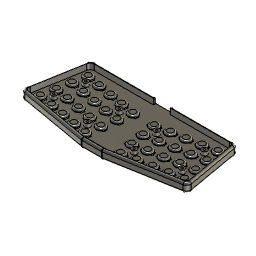
pusheenz40 low tolerance v2 v8 (Autodesk Fusion 360 design; units mm, degrees)
Autodesk Fusion 360 part; units mm, degrees
note: some values were not read from the file. Chosen so that the rebuilt part matches the saved one: which bodies a step acts on. Set by a fixed rule: which sketch regions a step uses.
(part 1 of 2)
sketch "Sketch1" plane through (0, 0, 0) normal (0, 0, 1) x (1, 0, 0)
  line L0 (-7.5882, -2.7237) -> (-0.9058, 35.1744)
  line L1 (2.0486, 37.6534) -> (102.6819, 37.6534)
  line L2 (105.6363, 35.1744) -> (112.3188, -2.7237)
  line L3 (109.8853, -6.1991) -> (59.9186, -15.0095)
  line L4 (59.3977, -15.0551) -> (45.3329, -15.0551)
  line L5 (44.8119, -15.0095) -> (-5.1548, -6.1991)
  arc A0 (2.0486, 37.6534) -> (-0.9058, 35.1744) centre (2.0486, 34.6534) ccw
  arc A1 (105.6363, 35.1744) -> (102.6819, 37.6534) centre (102.6819, 34.6534) ccw
  arc A2 (109.8853, -6.1991) -> (112.3188, -2.7237) centre (109.3644, -3.2446) ccw
  arc A3 (59.3977, -15.0551) -> (59.9186, -15.0095) centre (59.3977, -12.0551) ccw
  arc A4 (44.8119, -15.0095) -> (45.3329, -15.0551) centre (45.3329, -12.0551) ccw
  arc A5 (-7.5882, -2.7237) -> (-5.1548, -6.1991) centre (-4.6338, -3.2446) ccw
  line L6 (-5.8506, -1.507) -> (0.3109, 33.4367)
  line L7 (3.2654, 35.9157) -> (101.4652, 35.9157)
  line L8 (104.4196, 33.4367) -> (110.5811, -1.507)
  line L9 (108.1476, -4.9823) -> (61.1353, -13.2719)
  line L10 (60.6144, -13.3174) -> (44.1162, -13.3174)
  line L11 (43.5952, -13.2719) -> (-3.4171, -4.9823)
  arc A6 (3.2654, 35.9157) -> (0.3109, 33.4367) centre (3.2654, 32.9157) ccw
  arc A7 (104.4196, 33.4367) -> (101.4652, 35.9157) centre (101.4652, 32.9157) ccw
  arc A8 (108.1476, -4.9823) -> (110.5811, -1.507) centre (107.6267, -2.0279) ccw
  arc A9 (60.6144, -13.3174) -> (61.1353, -13.2719) centre (60.6144, -10.3174) ccw
  arc A10 (43.5952, -13.2719) -> (44.1162, -13.3174) centre (44.1162, -10.3174) ccw
  arc A11 (-5.8506, -1.507) -> (-3.4171, -4.9823) centre (-2.8961, -2.0279) ccw
  line L12 (-5.2713, -1.1014) -> (0.7165, 32.8575)
  line L13 (3.6709, 35.3365) -> (101.0596, 35.3365)
  line L14 (104.014, 32.8575) -> (110.0019, -1.1014)
  line L15 (107.5684, -4.5767) -> (61.5409, -12.6926)
  line L16 (61.02, -12.7382) -> (43.7106, -12.7382)
  line L17 (43.1896, -12.6926) -> (-2.8379, -4.5767)
  arc A12 (3.6709, 35.3365) -> (0.7165, 32.8575) centre (3.6709, 32.3365) ccw
  arc A13 (104.014, 32.8575) -> (101.0596, 35.3365) centre (101.0596, 32.3365) ccw
  arc A14 (107.5684, -4.5767) -> (110.0019, -1.1014) centre (107.0475, -1.6223) ccw
  arc A15 (61.02, -12.7382) -> (61.5409, -12.6926) centre (61.02, -9.7382) ccw
  arc A16 (43.1896, -12.6926) -> (43.7106, -12.7382) centre (43.7106, -9.7382) ccw
  arc A17 (-5.2713, -1.1014) -> (-2.8379, -4.5767) centre (-2.3169, -1.6223) ccw
  line L18 (-3.6888, -0.8219) -> (-3.3564, -0.8805)
  line L19 (2.8528, -1.9754) -> (3.1852, -2.034)
  arc A18 (3.1852, -2.034) -> (3.7644, -1.6284) centre (3.272, -1.5416) ccw
  line L20 (3.7644, -1.6284) -> (4.0943, 0.2427)
  arc A19 (4.0943, 0.2427) -> (3.6888, 0.8219) centre (3.6019, 0.3295) ccw
  line L21 (3.6888, 0.8219) -> (3.3564, 0.8805)
  line L22 (-2.8528, 1.9754) -> (-3.1852, 2.034)
  arc A20 (-3.1852, 2.034) -> (-3.7644, 1.6284) centre (-3.272, 1.5416) ccw
  line L23 (-3.7644, 1.6284) -> (-4.0943, -0.2427)
  arc A21 (-4.0943, -0.2427) -> (-3.6888, -0.8219) centre (-3.6019, -0.3295) ccw
  line L24 (-1.9523, 9.0261) -> (-1.6199, 8.9675)
  line L25 (4.5893, 7.8727) -> (4.9217, 7.8141)
  arc A22 (4.9217, 7.8141) -> (5.5009, 8.2197) centre (5.0085, 8.3065) ccw
  line L26 (5.5009, 8.2197) -> (5.8308, 10.0908)
  arc A23 (5.8308, 10.0908) -> (5.4253, 10.67) centre (5.3384, 10.1776) ccw
  line L27 (5.4253, 10.67) -> (5.0929, 10.7286)
  line L28 (-1.1164, 11.8235) -> (-1.4487, 11.8821)
  arc A24 (-1.4487, 11.8821) -> (-2.0279, 11.4765) centre (-1.5355, 11.3897) ccw
  line L29 (-2.0279, 11.4765) -> (-2.3579, 9.6054)
  arc A25 (-2.3579, 9.6054) -> (-1.9523, 9.0261) centre (-1.8655, 9.5185) ccw
  line L30 (-0.2158, 18.8742) -> (0.1165, 18.8156)
  line L31 (6.3258, 17.7208) -> (6.6582, 17.6622)
  arc A26 (6.6582, 17.6622) -> (7.2374, 18.0677) centre (6.745, 18.1546) ccw
  line L32 (7.2374, 18.0677) -> (7.5673, 19.9389)
  arc A27 (7.5673, 19.9389) -> (7.1617, 20.5181) centre (7.0749, 20.0257) ccw
  line L33 (7.1617, 20.5181) -> (6.8294, 20.5767)
  line L34 (0.6201, 21.6716) -> (0.2878, 21.7302)
  arc A28 (0.2878, 21.7302) -> (-0.2915, 21.3246) centre (0.201, 21.2378) ccw
  line L35 (-0.2915, 21.3246) -> (-0.6214, 19.4534)
  arc A29 (-0.6214, 19.4534) -> (-0.2158, 18.8742) centre (-0.129, 19.3666) ccw
  line L36 (1.5207, 28.7223) -> (1.853, 28.6637)
  line L37 (8.0623, 27.5688) -> (8.3946, 27.5102)
  arc A30 (8.3946, 27.5102) -> (8.9739, 27.9158) centre (8.4815, 28.0026) ccw
  line L38 (8.9739, 27.9158) -> (9.3038, 29.7869)
  arc A31 (9.3038, 29.7869) -> (8.8982, 30.3662) centre (8.8114, 29.8738) ccw
  line L39 (8.8982, 30.3662) -> (8.5659, 30.4248)
  line L40 (2.3566, 31.5196) -> (2.0243, 31.5782)
  arc A32 (2.0243, 31.5782) -> (1.445, 31.1727) centre (1.9374, 31.0858) ccw
  line L41 (1.445, 31.1727) -> (1.1151, 29.3015)
  arc A33 (1.1151, 29.3015) -> (1.5207, 28.7223) centre (1.6075, 29.2147) ccw
  line L42 (6.1593, -2.5584) -> (6.4917, -2.617)
  line L43 (12.7009, -3.7119) -> (13.0333, -3.7705)
  arc A34 (13.0333, -3.7705) -> (13.6125, -3.3649) centre (13.1201, -3.2781) ccw
  line L44 (13.6125, -3.3649) -> (13.9424, -1.4938)
  arc A35 (13.9424, -1.4938) -> (13.5368, -0.9145) centre (13.45, -1.4069) ccw
  line L45 (13.5368, -0.9145) -> (13.2045, -0.8559)
  line L46 (6.9952, 0.2389) -> (6.6629, 0.2975)
  arc A36 (6.6629, 0.2975) -> (6.0837, -0.1081) centre (6.5761, -0.1949) ccw
  line L47 (6.0837, -0.1081) -> (5.7537, -1.9792)
  arc A37 (5.7537, -1.9792) -> (6.1593, -2.5584) centre (6.2461, -2.066) ccw
  line L48 (7.8958, 7.2897) -> (8.2281, 7.2311)
  line L49 (14.4374, 6.1362) -> (14.7697, 6.0776)
  arc A38 (14.7697, 6.0776) -> (15.349, 6.4832) centre (14.8566, 6.57) ccw
  line L50 (15.349, 6.4832) -> (15.6789, 8.3543)
  arc A39 (15.6789, 8.3543) -> (15.2733, 8.9335) centre (15.1865, 8.4411) ccw
  line L51 (15.2733, 8.9335) -> (14.941, 8.9921)
  line L52 (8.7317, 10.087) -> (8.3994, 10.1456)
  arc A40 (8.3994, 10.1456) -> (7.8201, 9.74) centre (8.3125, 9.6532) ccw
  line L53 (7.8201, 9.74) -> (7.4902, 7.8689)
  arc A41 (7.4902, 7.8689) -> (7.8958, 7.2897) centre (7.9826, 7.7821) ccw
  line L54 (9.6323, 17.1377) -> (9.9646, 17.0791)
  line L55 (16.1739, 15.9843) -> (16.5062, 15.9257)
  arc A42 (16.5062, 15.9257) -> (17.0855, 16.3312) centre (16.5931, 16.4181) ccw
  line L56 (17.0855, 16.3312) -> (17.4154, 18.2024)
  arc A43 (17.4154, 18.2024) -> (17.0098, 18.7816) centre (16.923, 18.2892) ccw
  line L57 (17.0098, 18.7816) -> (16.6775, 18.8402)
  line L58 (10.4682, 19.9351) -> (10.1359, 19.9937)
  arc A44 (10.1359, 19.9937) -> (9.5566, 19.5881) centre (10.049, 19.5013) ccw
  line L59 (9.5566, 19.5881) -> (9.2267, 17.717)
  arc A45 (9.2267, 17.717) -> (9.6323, 17.1377) centre (9.7191, 17.6301) ccw
  line L60 (11.3688, 26.9858) -> (11.7011, 26.9272)
  line L61 (17.9104, 25.8323) -> (18.2427, 25.7737)
  arc A46 (18.2427, 25.7737) -> (18.8219, 26.1793) centre (18.3295, 26.2662) ccw
  line L62 (18.8219, 26.1793) -> (19.1519, 28.0505)
  arc A47 (19.1519, 28.0505) -> (18.7463, 28.6297) centre (18.6595, 28.1373) ccw
  line L63 (18.7463, 28.6297) -> (18.4139, 28.6883)
  line L64 (12.2047, 29.7832) -> (11.8723, 29.8418)
  arc A48 (11.8723, 29.8418) -> (11.2931, 29.4362) centre (11.7855, 29.3494) ccw
  line L65 (11.2931, 29.4362) -> (10.9632, 27.565)
  arc A49 (10.9632, 27.565) -> (11.3688, 26.9858) centre (11.4556, 27.4782) ccw
  line L66 (16.0074, -4.2949) -> (16.3397, -4.3535)
  line L67 (22.549, -5.4484) -> (22.8813, -5.507)
  arc A50 (22.8813, -5.507) -> (23.4606, -5.1014) centre (22.9682, -5.0146) ccw
  line L68 (23.4606, -5.1014) -> (23.7905, -3.2303)
  arc A51 (23.7905, -3.2303) -> (23.3849, -2.651) centre (23.2981, -3.1434) ccw
  line L69 (23.3849, -2.651) -> (23.0526, -2.5924)
  line L70 (16.8433, -1.4976) -> (16.511, -1.439)
  arc A52 (16.511, -1.439) -> (15.9317, -1.8445) centre (16.4241, -1.9314) ccw
  line L71 (15.9317, -1.8445) -> (15.6018, -3.7157)
  arc A53 (15.6018, -3.7157) -> (16.0074, -4.2949) centre (16.0942, -3.8025) ccw
  line L72 (17.7439, 5.5532) -> (18.0762, 5.4946)
  line L73 (24.2855, 4.3997) -> (24.6178, 4.3411)
  arc A54 (24.6178, 4.3411) -> (25.1971, 4.7467) centre (24.7047, 4.8335) ccw
  line L74 (25.1971, 4.7467) -> (25.527, 6.6178)
  arc A55 (25.527, 6.6178) -> (25.1214, 7.1971) centre (25.0346, 6.7046) ccw
  line L75 (25.1214, 7.1971) -> (24.7891, 7.2557)
  line L76 (18.5798, 8.3505) -> (18.2474, 8.4091)
  arc A56 (18.2474, 8.4091) -> (17.6682, 8.0035) centre (18.1606, 7.9167) ccw
  line L77 (17.6682, 8.0035) -> (17.3383, 6.1324)
  arc A57 (17.3383, 6.1324) -> (17.7439, 5.5532) centre (17.8307, 6.0456) ccw
  line L78 (19.4803, 15.4013) -> (19.8127, 15.3427)
  line L79 (26.022, 14.2478) -> (26.3543, 14.1892)
  arc A58 (26.3543, 14.1892) -> (26.9335, 14.5948) centre (26.4411, 14.6816) ccw
  line L80 (26.9335, 14.5948) -> (27.2635, 16.4659)
  arc A59 (27.2635, 16.4659) -> (26.8579, 17.0451) centre (26.7711, 16.5527) ccw
  line L81 (26.8579, 17.0451) -> (26.5255, 17.1037)
  line L82 (20.3163, 18.1986) -> (19.9839, 18.2572)
  arc A60 (19.9839, 18.2572) -> (19.4047, 17.8516) centre (19.8971, 17.7648) ccw
  line L83 (19.4047, 17.8516) -> (19.0748, 15.9805)
  arc A61 (19.0748, 15.9805) -> (19.4803, 15.4013) centre (19.5672, 15.8937) ccw
  line L84 (21.2168, 25.2493) -> (21.5492, 25.1907)
  line L85 (27.7584, 24.0959) -> (28.0908, 24.0373)
  arc A62 (28.0908, 24.0373) -> (28.67, 24.4428) centre (28.1776, 24.5297) ccw
  line L86 (28.67, 24.4428) -> (28.9999, 26.314)
  arc A63 (28.9999, 26.314) -> (28.5944, 26.8932) centre (28.5075, 26.4008) ccw
  line L87 (28.5944, 26.8932) -> (28.262, 26.9518)
  line L88 (22.0528, 28.0467) -> (21.7204, 28.1053)
  arc A64 (21.7204, 28.1053) -> (21.1412, 27.6997) centre (21.6336, 27.6129) ccw
  line L89 (21.1412, 27.6997) -> (20.8113, 25.8286)
  arc A65 (20.8113, 25.8286) -> (21.2168, 25.2493) centre (21.3037, 25.7417) ccw
  line L90 (25.8555, -6.0314) -> (26.1878, -6.09)
  line L91 (32.3971, -7.1848) -> (32.7294, -7.2434)
  arc A66 (32.7294, -7.2434) -> (33.3086, -6.8379) centre (32.8162, -6.751) ccw
  line L92 (33.3086, -6.8379) -> (33.6386, -4.9667)
  arc A67 (33.6386, -4.9667) -> (33.233, -4.3875) centre (33.1462, -4.8799) ccw
  line L93 (33.233, -4.3875) -> (32.9007, -4.3289)
  line L94 (26.6914, -3.234) -> (26.359, -3.1754)
  arc A68 (26.359, -3.1754) -> (25.7798, -3.581) centre (26.2722, -3.6678) ccw
  line L95 (25.7798, -3.581) -> (25.4499, -5.4522)
  arc A69 (25.4499, -5.4522) -> (25.8555, -6.0314) centre (25.9423, -5.539) ccw
  line L96 (27.5919, 3.8167) -> (27.9243, 3.7581)
  line L97 (34.1336, 2.6632) -> (34.4659, 2.6046)
  arc A70 (34.4659, 2.6046) -> (35.0451, 3.0102) centre (34.5527, 3.097) ccw
  line L98 (35.0451, 3.0102) -> (35.3751, 4.8813)
  arc A71 (35.3751, 4.8813) -> (34.9695, 5.4606) centre (34.8827, 4.9682) ccw
  line L99 (34.9695, 5.4606) -> (34.6371, 5.5192)
  line L100 (28.4279, 6.614) -> (28.0955, 6.6726)
  arc A72 (28.0955, 6.6726) -> (27.5163, 6.2671) centre (28.0087, 6.1802) ccw
  line L101 (27.5163, 6.2671) -> (27.1864, 4.3959)
  arc A73 (27.1864, 4.3959) -> (27.5919, 3.8167) centre (27.6788, 4.3091) ccw
  line L102 (29.3284, 13.6648) -> (29.6608, 13.6062)
  line L103 (35.87, 12.5113) -> (36.2024, 12.4527)
  arc A74 (36.2024, 12.4527) -> (36.7816, 12.8583) centre (36.2892, 12.9451) ccw
  line L104 (36.7816, 12.8583) -> (37.1115, 14.7294)
  arc A75 (37.1115, 14.7294) -> (36.706, 15.3086) centre (36.6191, 14.8162) ccw
  line L105 (36.706, 15.3086) -> (36.3736, 15.3673)
  line L106 (30.1644, 16.4621) -> (29.832, 16.5207)
  arc A76 (29.832, 16.5207) -> (29.2528, 16.1151) centre (29.7452, 16.0283) ccw
  line L107 (29.2528, 16.1151) -> (28.9228, 14.244)
  arc A77 (28.9228, 14.244) -> (29.3284, 13.6648) centre (29.4153, 14.1572) ccw
  line L108 (31.0649, 23.5128) -> (31.3973, 23.4542)
  line L109 (37.6065, 22.3594) -> (37.9389, 22.3008)
  arc A78 (37.9389, 22.3008) -> (38.5181, 22.7064) centre (38.0257, 22.7932) ccw
  line L110 (38.5181, 22.7064) -> (38.848, 24.5775)
  arc A79 (38.848, 24.5775) -> (38.4424, 25.1567) centre (38.3556, 24.6643) ccw
  line L111 (38.4424, 25.1567) -> (38.1101, 25.2153)
  line L112 (31.9008, 26.3102) -> (31.5685, 26.3688)
  arc A80 (31.5685, 26.3688) -> (30.9893, 25.9632) centre (31.4817, 25.8764) ccw
  line L113 (30.9893, 25.9632) -> (30.6593, 24.0921)
  arc A81 (30.6593, 24.0921) -> (31.0649, 23.5128) centre (31.1517, 24.0053) ccw
  line L114 (35.7035, -7.7679) -> (36.0359, -7.8265)
  line L115 (42.2451, -8.9213) -> (42.5775, -8.9799)
  arc A82 (42.5775, -8.9799) -> (43.1567, -8.5744) centre (42.6643, -8.4875) ccw
  line L116 (43.1567, -8.5744) -> (43.4867, -6.7032)
  arc A83 (43.4867, -6.7032) -> (43.0811, -6.124) centre (42.9943, -6.6164) ccw
  line L117 (43.0811, -6.124) -> (42.7487, -6.0654)
  line L118 (36.5395, -4.9705) -> (36.2071, -4.9119)
  arc A84 (36.2071, -4.9119) -> (35.6279, -5.3175) centre (36.1203, -5.4043) ccw
  line L119 (35.6279, -5.3175) -> (35.298, -7.1886)
  arc A85 (35.298, -7.1886) -> (35.7035, -7.7679) centre (35.7904, -7.2755) ccw
  line L120 (37.44, 2.0802) -> (37.7724, 2.0216)
  line L121 (43.9816, 0.9267) -> (44.314, 0.8681)
  arc A86 (44.314, 0.8681) -> (44.8932, 1.2737) centre (44.4008, 1.3606) ccw
  line L122 (44.8932, 1.2737) -> (45.2231, 3.1449)
  arc A87 (45.2231, 3.1449) -> (44.8176, 3.7241) centre (44.7307, 3.2317) ccw
  line L123 (44.8176, 3.7241) -> (44.4852, 3.7827)
  line L124 (38.276, 4.8776) -> (37.9436, 4.9362)
  arc A88 (37.9436, 4.9362) -> (37.3644, 4.5306) centre (37.8568, 4.4437) ccw
  line L125 (37.3644, 4.5306) -> (37.0344, 2.6594)
  arc A89 (37.0344, 2.6594) -> (37.44, 2.0802) centre (37.5268, 2.5726) ccw
  line L126 (39.1765, 11.9283) -> (39.5089, 11.8697)
  line L127 (45.7181, 10.7748) -> (46.0505, 10.7162)
  arc A90 (46.0505, 10.7162) -> (46.6297, 11.1218) centre (46.1373, 11.2086) ccw
  line L128 (46.6297, 11.1218) -> (46.9596, 12.9929)
  arc A91 (46.9596, 12.9929) -> (46.554, 13.5722) centre (46.4672, 13.0798) ccw
  line L129 (46.554, 13.5722) -> (46.2217, 13.6308)
  line L130 (40.0124, 14.7256) -> (39.6801, 14.7842)
  arc A92 (39.6801, 14.7842) -> (39.1009, 14.3787) centre (39.5933, 14.2918) ccw
  line L131 (39.1009, 14.3787) -> (38.7709, 12.5075)
  arc A93 (38.7709, 12.5075) -> (39.1765, 11.9283) centre (39.2633, 12.4207) ccw
  line L132 (40.913, 21.7764) -> (41.2453, 21.7178)
  line L133 (47.4546, 20.6229) -> (47.7869, 20.5643)
  arc A94 (47.7869, 20.5643) -> (48.3662, 20.9699) centre (47.8738, 21.0567) ccw
  line L134 (48.3662, 20.9699) -> (48.6961, 22.841)
  arc A95 (48.6961, 22.841) -> (48.2905, 23.4202) centre (48.2037, 22.9278) ccw
  line L135 (48.2905, 23.4202) -> (47.9582, 23.4788)
  line L136 (41.7489, 24.5737) -> (41.4166, 24.6323)
  arc A96 (41.4166, 24.6323) -> (40.8373, 24.2267) centre (41.3297, 24.1399) ccw
  line L137 (40.8373, 24.2267) -> (40.5074, 22.3556)
  arc A97 (40.5074, 22.3556) -> (40.913, 21.7764) centre (40.9998, 22.2688) ccw
  line L138 (101.5454, -2.034) -> (101.8777, -1.9754)
  line L139 (108.087, -0.8805) -> (108.4193, -0.8219)
  arc A98 (108.4193, -0.8219) -> (108.8249, -0.2427) centre (108.3325, -0.3295) ccw
  line L140 (108.8249, -0.2427) -> (108.495, 1.6284)
  arc A99 (108.495, 1.6284) -> (107.9157, 2.034) centre (108.0026, 1.5416) ccw
  line L141 (107.9157, 2.034) -> (107.5834, 1.9754)
  line L142 (101.3741, 0.8805) -> (101.0418, 0.8219)
  arc A100 (101.0418, 0.8219) -> (100.6362, 0.2427) centre (101.1286, 0.3295) ccw
  line L143 (100.6362, 0.2427) -> (100.9661, -1.6284)
  arc A101 (100.9661, -1.6284) -> (101.5454, -2.034) centre (101.4585, -1.5416) ccw
  line L144 (99.8089, 7.8141) -> (100.1412, 7.8727)
  line L145 (106.3505, 8.9675) -> (106.6828, 9.0261)
  arc A102 (106.6828, 9.0261) -> (107.0884, 9.6054) centre (106.596, 9.5185) ccw
  line L146 (107.0884, 9.6054) -> (106.7585, 11.4765)
  arc A103 (106.7585, 11.4765) -> (106.1793, 11.8821) centre (106.2661, 11.3897) ccw
  line L147 (106.1793, 11.8821) -> (105.8469, 11.8235)
  line L148 (99.6376, 10.7286) -> (99.3053, 10.67)
  arc A104 (99.3053, 10.67) -> (98.8997, 10.0908) centre (99.3921, 10.1776) ccw
  line L149 (98.8997, 10.0908) -> (99.2296, 8.2197)
  arc A105 (99.2296, 8.2197) -> (99.8089, 7.8141) centre (99.7221, 8.3065) ccw
  line L150 (98.0724, 17.6622) -> (98.4047, 17.7208)
  line L151 (104.614, 18.8156) -> (104.9464, 18.8742)
  arc A106 (104.9464, 18.8742) -> (105.3519, 19.4534) centre (104.8595, 19.3666) ccw
  line L152 (105.3519, 19.4534) -> (105.022, 21.3246)
  arc A107 (105.022, 21.3246) -> (104.4428, 21.7302) centre (104.5296, 21.2378) ccw
  line L153 (104.4428, 21.7302) -> (104.1104, 21.6716)
  line L154 (97.9012, 20.5767) -> (97.5688, 20.5181)
  arc A108 (97.5688, 20.5181) -> (97.1632, 19.9389) centre (97.6556, 20.0257) ccw
  line L155 (97.1632, 19.9389) -> (97.4932, 18.0677)
  arc A109 (97.4932, 18.0677) -> (98.0724, 17.6622) centre (97.9856, 18.1546) ccw
  line L156 (96.3359, 27.5102) -> (96.6683, 27.5688)
  line L157 (102.8775, 28.6637) -> (103.2099, 28.7223)
  arc A110 (103.2099, 28.7223) -> (103.6155, 29.3015) centre (103.123, 29.2147) ccw
  line L158 (103.6155, 29.3015) -> (103.2855, 31.1727)
  arc A111 (103.2855, 31.1727) -> (102.7063, 31.5782) centre (102.7931, 31.0858) ccw
  line L159 (102.7063, 31.5782) -> (102.3739, 31.5196)
  line L160 (96.1647, 30.4248) -> (95.8323, 30.3662)
  arc A112 (95.8323, 30.3662) -> (95.4268, 29.7869) centre (95.9192, 29.8738) ccw
  line L161 (95.4268, 29.7869) -> (95.7567, 27.9158)
  arc A113 (95.7567, 27.9158) -> (96.3359, 27.5102) centre (96.2491, 28.0026) ccw
  line L162 (91.6973, -3.7705) -> (92.0296, -3.7119)
  line L163 (98.2389, -2.617) -> (98.5712, -2.5584)
  arc A114 (98.5712, -2.5584) -> (98.9768, -1.9792) centre (98.4844, -2.066) ccw
  line L164 (98.9768, -1.9792) -> (98.6469, -0.1081)
  arc A115 (98.6469, -0.1081) -> (98.0677, 0.2975) centre (98.1545, -0.1949) ccw
  line L165 (98.0677, 0.2975) -> (97.7353, 0.2389)
  line L166 (91.5261, -0.8559) -> (91.1937, -0.9145)
  arc A116 (91.1937, -0.9145) -> (90.7881, -1.4938) centre (91.2805, -1.4069) ccw
  line L167 (90.7881, -1.4938) -> (91.1181, -3.3649)
  arc A117 (91.1181, -3.3649) -> (91.6973, -3.7705) centre (91.6105, -3.2781) ccw
  line L168 (89.9608, 6.0776) -> (90.2931, 6.1362)
  line L169 (96.5024, 7.2311) -> (96.8348, 7.2897)
  arc A118 (96.8348, 7.2897) -> (97.2403, 7.8689) centre (96.7479, 7.7821) ccw
  line L170 (97.2403, 7.8689) -> (96.9104, 9.74)
  arc A119 (96.9104, 9.74) -> (96.3312, 10.1456) centre (96.418, 9.6532) ccw
  line L171 (96.3312, 10.1456) -> (95.9988, 10.087)
  line L172 (89.7896, 8.9921) -> (89.4572, 8.9335)
  arc A120 (89.4572, 8.9335) -> (89.0516, 8.3543) centre (89.544, 8.4411) ccw
  line L173 (89.0516, 8.3543) -> (89.3816, 6.4832)
  arc A121 (89.3816, 6.4832) -> (89.9608, 6.0776) centre (89.874, 6.57) ccw
  line L174 (88.2243, 15.9257) -> (88.5567, 15.9843)
  line L175 (94.7659, 17.0791) -> (95.0983, 17.1377)
  arc A122 (95.0983, 17.1377) -> (95.5039, 17.717) centre (95.0115, 17.6301) ccw
  line L176 (95.5039, 17.717) -> (95.1739, 19.5881)
  arc A123 (95.1739, 19.5881) -> (94.5947, 19.9937) centre (94.6815, 19.5013) ccw
  line L177 (94.5947, 19.9937) -> (94.2623, 19.9351)
  line L178 (88.0531, 18.8402) -> (87.7207, 18.7816)
  arc A124 (87.7207, 18.7816) -> (87.3152, 18.2024) centre (87.8076, 18.2892) ccw
  line L179 (87.3152, 18.2024) -> (87.6451, 16.3312)
  arc A125 (87.6451, 16.3312) -> (88.2243, 15.9257) centre (88.1375, 16.4181) ccw
  line L180 (86.4878, 25.7737) -> (86.8202, 25.8323)
  line L181 (93.0294, 26.9272) -> (93.3618, 26.9858)
  arc A126 (93.3618, 26.9858) -> (93.7674, 27.565) centre (93.275, 27.4782) ccw
  line L182 (93.7674, 27.565) -> (93.4374, 29.4362)
  arc A127 (93.4374, 29.4362) -> (92.8582, 29.8418) centre (92.945, 29.3494) ccw
  line L183 (92.8582, 29.8418) -> (92.5259, 29.7832)
  line L184 (86.3166, 28.6883) -> (85.9843, 28.6297)
  arc A128 (85.9843, 28.6297) -> (85.5787, 28.0505) centre (86.0711, 28.1373) ccw
  line L185 (85.5787, 28.0505) -> (85.9086, 26.1793)
  arc A129 (85.9086, 26.1793) -> (86.4878, 25.7737) centre (86.401, 26.2662) ccw
  line L186 (81.8492, -5.507) -> (82.1816, -5.4484)
  line L187 (88.3908, -4.3535) -> (88.7232, -4.2949)
  arc A130 (88.7232, -4.2949) -> (89.1287, -3.7157) centre (88.6363, -3.8025) ccw
  line L188 (89.1287, -3.7157) -> (88.7988, -1.8445)
  arc A131 (88.7988, -1.8445) -> (88.2196, -1.439) centre (88.3064, -1.9314) ccw
  line L189 (88.2196, -1.439) -> (87.8872, -1.4976)
  line L190 (81.678, -2.5924) -> (81.3456, -2.651)
  arc A132 (81.3456, -2.651) -> (80.94, -3.2303) centre (81.4324, -3.1434) ccw
  line L191 (80.94, -3.2303) -> (81.27, -5.1014)
  arc A133 (81.27, -5.1014) -> (81.8492, -5.507) centre (81.7624, -5.0146) ccw
  line L192 (80.1127, 4.3411) -> (80.4451, 4.3997)
  line L193 (86.6543, 5.4946) -> (86.9867, 5.5532)
  arc A134 (86.9867, 5.5532) -> (87.3923, 6.1324) centre (86.8999, 6.0456) ccw
  line L194 (87.3923, 6.1324) -> (87.0623, 8.0035)
  arc A135 (87.0623, 8.0035) -> (86.4831, 8.4091) centre (86.5699, 7.9167) ccw
  line L195 (86.4831, 8.4091) -> (86.1507, 8.3505)
  line L196 (79.9415, 7.2557) -> (79.6091, 7.1971)
  arc A136 (79.6091, 7.1971) -> (79.2036, 6.6178) centre (79.696, 6.7046) ccw
  line L197 (79.2036, 6.6178) -> (79.5335, 4.7467)
  arc A137 (79.5335, 4.7467) -> (80.1127, 4.3411) centre (80.0259, 4.8335) ccw
  line L198 (78.3762, 14.1892) -> (78.7086, 14.2478)
  line L199 (84.9178, 15.3427) -> (85.2502, 15.4013)
  arc A138 (85.2502, 15.4013) -> (85.6558, 15.9805) centre (85.1634, 15.8937) ccw
  line L200 (85.6558, 15.9805) -> (85.3258, 17.8516)
  arc A139 (85.3258, 17.8516) -> (84.7466, 18.2572) centre (84.8334, 17.7648) ccw
  line L201 (84.7466, 18.2572) -> (84.4143, 18.1986)
  line L202 (78.205, 17.1037) -> (77.8727, 17.0451)
  arc A140 (77.8727, 17.0451) -> (77.4671, 16.4659) centre (77.9595, 16.5527) ccw
  line L203 (77.4671, 16.4659) -> (77.797, 14.5948)
  arc A141 (77.797, 14.5948) -> (78.3762, 14.1892) centre (78.2894, 14.6816) ccw
  line L204 (76.6398, 24.0373) -> (76.9721, 24.0959)
  line L205 (83.1814, 25.1907) -> (83.5137, 25.2493)
  arc A142 (83.5137, 25.2493) -> (83.9193, 25.8286) centre (83.4269, 25.7417) ccw
  line L206 (83.9193, 25.8286) -> (83.5894, 27.6997)
  arc A143 (83.5894, 27.6997) -> (83.0101, 28.1053) centre (83.097, 27.6129) ccw
  line L207 (83.0101, 28.1053) -> (82.6778, 28.0467)
  line L208 (76.4685, 26.9518) -> (76.1362, 26.8932)
  arc A144 (76.1362, 26.8932) -> (75.7306, 26.314) centre (76.223, 26.4008) ccw
  line L209 (75.7306, 26.314) -> (76.0605, 24.4428)
  arc A145 (76.0605, 24.4428) -> (76.6398, 24.0373) centre (76.5529, 24.5297) ccw
  line L210 (72.0011, -7.2434) -> (72.3335, -7.1848)
  line L211 (78.5427, -6.09) -> (78.8751, -6.0314)
  arc A146 (78.8751, -6.0314) -> (79.2807, -5.4522) centre (78.7883, -5.539) ccw
  line L212 (79.2807, -5.4522) -> (78.9507, -3.581)
  arc A147 (78.9507, -3.581) -> (78.3715, -3.1754) centre (78.4583, -3.6678) ccw
  line L213 (78.3715, -3.1754) -> (78.0392, -3.234)
  line L214 (71.8299, -4.3289) -> (71.4975, -4.3875)
  arc A148 (71.4975, -4.3875) -> (71.092, -4.9667) centre (71.5844, -4.8799) ccw
  line L215 (71.092, -4.9667) -> (71.4219, -6.8379)
  arc A149 (71.4219, -6.8379) -> (72.0011, -7.2434) centre (71.9143, -6.751) ccw
  line L216 (70.2646, 2.6046) -> (70.597, 2.6632)
  line L217 (76.8063, 3.7581) -> (77.1386, 3.8167)
  arc A150 (77.1386, 3.8167) -> (77.5442, 4.3959) centre (77.0518, 4.3091) ccw
  line L218 (77.5442, 4.3959) -> (77.2143, 6.2671)
  arc A151 (77.2143, 6.2671) -> (76.635, 6.6726) centre (76.7218, 6.1802) ccw
  line L219 (76.635, 6.6726) -> (76.3027, 6.614)
  line L220 (70.0934, 5.5192) -> (69.7611, 5.4606)
  arc A152 (69.7611, 5.4606) -> (69.3555, 4.8813) centre (69.8479, 4.9682) ccw
  line L221 (69.3555, 4.8813) -> (69.6854, 3.0102)
  arc A153 (69.6854, 3.0102) -> (70.2646, 2.6046) centre (70.1778, 3.097) ccw
  line L222 (68.5282, 12.4527) -> (68.8605, 12.5113)
  line L223 (75.0698, 13.6062) -> (75.4021, 13.6648)
  arc A154 (75.4021, 13.6648) -> (75.8077, 14.244) centre (75.3153, 14.1572) ccw
  line L224 (75.8077, 14.244) -> (75.4778, 16.1151)
  arc A155 (75.4778, 16.1151) -> (74.8985, 16.5207) centre (74.9854, 16.0283) ccw
  line L225 (74.8985, 16.5207) -> (74.5662, 16.4621)
  line L226 (68.3569, 15.3673) -> (68.0246, 15.3086)
  arc A156 (68.0246, 15.3086) -> (67.619, 14.7294) centre (68.1114, 14.8162) ccw
  line L227 (67.619, 14.7294) -> (67.9489, 12.8583)
  arc A157 (67.9489, 12.8583) -> (68.5282, 12.4527) centre (68.4413, 12.9451) ccw
  line L228 (66.7917, 22.3008) -> (67.124, 22.3594)
  line L229 (73.3333, 23.4542) -> (73.6656, 23.5128)
  arc A158 (73.6656, 23.5128) -> (74.0712, 24.0921) centre (73.5788, 24.0053) ccw
  line L230 (74.0712, 24.0921) -> (73.7413, 25.9632)
  arc A159 (73.7413, 25.9632) -> (73.1621, 26.3688) centre (73.2489, 25.8764) ccw
  line L231 (73.1621, 26.3688) -> (72.8297, 26.3102)
  line L232 (66.6205, 25.2153) -> (66.2881, 25.1567)
  arc A160 (66.2881, 25.1567) -> (65.8825, 24.5775) centre (66.3749, 24.6643) ccw
  line L233 (65.8825, 24.5775) -> (66.2125, 22.7064)
  arc A161 (66.2125, 22.7064) -> (66.7917, 22.3008) centre (66.7049, 22.7932) ccw
  line L234 (62.153, -8.9799) -> (62.4854, -8.9213)
  line L235 (68.6947, -7.8265) -> (69.027, -7.7679)
  arc A162 (69.027, -7.7679) -> (69.4326, -7.1886) centre (68.9402, -7.2755) ccw
  line L236 (69.4326, -7.1886) -> (69.1027, -5.3175)
  arc A163 (69.1027, -5.3175) -> (68.5234, -4.9119) centre (68.6103, -5.4043) ccw
  line L237 (68.5234, -4.9119) -> (68.1911, -4.9705)
  line L238 (61.9818, -6.0654) -> (61.6495, -6.124)
  arc A164 (61.6495, -6.124) -> (61.2439, -6.7032) centre (61.7363, -6.6164) ccw
  line L239 (61.2439, -6.7032) -> (61.5738, -8.5744)
  arc A165 (61.5738, -8.5744) -> (62.153, -8.9799) centre (62.0662, -8.4875) ccw
  line L240 (60.4166, 0.8681) -> (60.7489, 0.9267)
  line L241 (66.9582, 2.0216) -> (67.2905, 2.0802)
  arc A166 (67.2905, 2.0802) -> (67.6961, 2.6594) centre (67.2037, 2.5726) ccw
  line L242 (67.6961, 2.6594) -> (67.3662, 4.5306)
  arc A167 (67.3662, 4.5306) -> (66.7869, 4.9362) centre (66.8738, 4.4437) ccw
  line L243 (66.7869, 4.9362) -> (66.4546, 4.8776)
  line L244 (60.2453, 3.7827) -> (59.913, 3.7241)
  arc A168 (59.913, 3.7241) -> (59.5074, 3.1449) centre (59.9998, 3.2317) ccw
  line L245 (59.5074, 3.1449) -> (59.8373, 1.2737)
  arc A169 (59.8373, 1.2737) -> (60.4166, 0.8681) centre (60.3297, 1.3606) ccw
  line L246 (58.6801, 10.7162) -> (59.0124, 10.7748)
  line L247 (65.2217, 11.8697) -> (65.554, 11.9283)
  arc A170 (65.554, 11.9283) -> (65.9596, 12.5075) centre (65.4672, 12.4207) ccw
  line L248 (65.9596, 12.5075) -> (65.6297, 14.3787)
  arc A171 (65.6297, 14.3787) -> (65.0505, 14.7842) centre (65.1373, 14.2918) ccw
  line L249 (65.0505, 14.7842) -> (64.7181, 14.7256)
  line L250 (58.5089, 13.6308) -> (58.1765, 13.5722)
  arc A172 (58.1765, 13.5722) -> (57.7709, 12.9929) centre (58.2633, 13.0798) ccw
  line L251 (57.7709, 12.9929) -> (58.1009, 11.1218)
  arc A173 (58.1009, 11.1218) -> (58.6801, 10.7162) centre (58.5933, 11.2086) ccw
  line L252 (56.9436, 20.5643) -> (57.276, 20.6229)
  line L253 (63.4852, 21.7178) -> (63.8176, 21.7764)
  arc A174 (63.8176, 21.7764) -> (64.2231, 22.3556) centre (63.7307, 22.2688) ccw
  line L254 (64.2231, 22.3556) -> (63.8932, 24.2267)
  arc A175 (63.8932, 24.2267) -> (63.314, 24.6323) centre (63.4008, 24.1399) ccw
  line L255 (63.314, 24.6323) -> (62.9816, 24.5737)
  line L256 (56.7724, 23.4788) -> (56.44, 23.4202)
  arc A176 (56.44, 23.4202) -> (56.0344, 22.841) centre (56.5268, 22.9278) ccw
  line L257 (56.0344, 22.841) -> (56.3644, 20.9699)
  arc A177 (56.3644, 20.9699) -> (56.9436, 20.5643) centre (56.8568, 21.0567) ccw
  arc A178 (-2.8528, 1.9754) -> (-2.8528, 1.9754) centre (0, 0) ccw
  arc A179 (-1.1164, 11.8235) -> (-1.1164, 11.8235) centre (1.7365, 9.8481) ccw
  arc A180 (0.6201, 21.6716) -> (0.6201, 21.6716) centre (3.473, 19.6962) ccw
  arc A181 (2.3566, 31.5196) -> (2.3566, 31.5196) centre (5.2094, 29.5442) ccw
  arc A182 (6.9952, 0.2389) -> (6.9952, 0.2389) centre (9.8481, -1.7365) ccw
  arc A183 (8.7317, 10.087) -> (8.7317, 10.087) centre (11.5846, 8.1116) ccw
  arc A184 (10.4682, 19.9351) -> (10.4682, 19.9351) centre (13.321, 17.9597) ccw
  arc A185 (12.2047, 29.7832) -> (12.2047, 29.7832) centre (15.0575, 27.8078) ccw
  arc A186 (16.8433, -1.4976) -> (16.8433, -1.4976) centre (19.6962, -3.473) ccw
  arc A187 (18.5798, 8.3505) -> (18.5798, 8.3505) centre (21.4326, 6.3751) ccw
  arc A188 (20.3163, 18.1986) -> (20.3163, 18.1986) centre (23.1691, 16.2232) ccw
  arc A189 (22.0528, 28.0467) -> (22.0528, 28.0467) centre (24.9056, 26.0713) ccw
  arc A190 (26.6914, -3.234) -> (26.6914, -3.234) centre (29.5442, -5.2094) ccw
  arc A191 (28.4279, 6.614) -> (28.4279, 6.614) centre (31.2807, 4.6386) ccw
  arc A192 (30.1644, 16.4621) -> (30.1644, 16.4621) centre (33.0172, 14.4867) ccw
  arc A193 (31.9008, 26.3102) -> (31.9008, 26.3102) centre (34.7537, 24.3348) ccw
  arc A194 (36.5395, -4.9705) -> (36.5395, -4.9705) centre (39.3923, -6.9459) ccw
  arc A195 (38.276, 4.8776) -> (38.276, 4.8776) centre (41.1288, 2.9022) ccw
  arc A196 (40.0124, 14.7256) -> (40.0124, 14.7256) centre (42.8653, 12.7502) ccw
  arc A197 (41.7489, 24.5737) -> (41.7489, 24.5737) centre (44.6018, 22.5983) ccw
  arc A198 (101.3741, 0.8805) -> (101.3741, 0.8805) centre (104.7305, 0) ccw
  arc A199 (99.6376, 10.7286) -> (99.6376, 10.7286) centre (102.9941, 9.8481) ccw
  arc A200 (97.9012, 20.5767) -> (97.9012, 20.5767) centre (101.2576, 19.6962) ccw
  arc A201 (96.1647, 30.4248) -> (96.1647, 30.4248) centre (99.5211, 29.5442) ccw
  arc A202 (91.5261, -0.8559) -> (91.5261, -0.8559) centre (94.8825, -1.7365) ccw
  arc A203 (89.7896, 8.9921) -> (89.7896, 8.9921) centre (93.146, 8.1116) ccw
  arc A204 (88.0531, 18.8402) -> (88.0531, 18.8402) centre (91.4095, 17.9597) ccw
  arc A205 (86.3166, 28.6883) -> (86.3166, 28.6883) centre (89.673, 27.8078) ccw
  arc A206 (81.678, -2.5924) -> (81.678, -2.5924) centre (85.0344, -3.473) ccw
  arc A207 (79.9415, 7.2557) -> (79.9415, 7.2557) centre (83.2979, 6.3751) ccw
  arc A208 (78.205, 17.1037) -> (78.205, 17.1037) centre (81.5614, 16.2232) ccw
  arc A209 (76.4685, 26.9518) -> (76.4685, 26.9518) centre (79.8249, 26.0713) ccw
  arc A210 (71.8299, -4.3289) -> (71.8299, -4.3289) centre (75.1863, -5.2094) ccw
  arc A211 (70.0934, 5.5192) -> (70.0934, 5.5192) centre (73.4498, 4.6386) ccw
  arc A212 (68.3569, 15.3673) -> (68.3569, 15.3673) centre (71.7134, 14.4867) ccw
  arc A213 (66.6205, 25.2153) -> (66.6205, 25.2153) centre (69.9769, 24.3348) ccw
  arc A214 (61.9818, -6.0654) -> (61.9818, -6.0654) centre (65.3382, -6.9459) ccw
  arc A215 (60.2453, 3.7827) -> (60.2453, 3.7827) centre (63.6018, 2.9022) ccw
  arc A216 (58.5089, 13.6308) -> (58.5089, 13.6308) centre (61.8653, 12.7502) ccw
  arc A217 (56.7724, 23.4788) -> (56.7724, 23.4788) centre (60.1288, 22.5983) ccw
  circle A218 centre (5.7923, 4.0558) radius 2
  circle A219 centre (9.2652, 23.752) radius 2
  circle A220 centre (35.3365, -1.1536) radius 2
  circle A221 centre (38.8095, 18.5425) radius 2
  circle A222 centre (98.9383, 4.0558) radius 2
  circle A223 centre (95.4653, 23.752) radius 2
  circle A224 centre (69.394, -1.1536) radius 2
  circle A225 centre (65.9211, 18.5425) radius 2
  circle A226 centre (5.7923, 4.0558) radius 0.75
  circle A227 centre (9.2652, 23.752) radius 0.75
  circle A228 centre (35.3365, -1.1536) radius 0.75
  circle A229 centre (38.8095, 18.5425) radius 0.75
  circle A230 centre (98.9383, 4.0558) radius 0.75
  circle A231 centre (95.4653, 23.752) radius 0.75
  circle A232 centre (69.394, -1.1536) radius 0.75
  circle A233 centre (65.9211, 18.5425) radius 0.75
  circle A234 centre (0, 0) radius 3.47
  circle A235 centre (1.7365, 9.8481) radius 3.47
  circle A236 centre (3.473, 19.6962) radius 3.47
  circle A237 centre (5.2094, 29.5442) radius 3.47
  circle A238 centre (15.0575, 27.8078) radius 3.47
  circle A239 centre (13.321, 17.9597) radius 3.47
  circle A240 centre (11.5846, 8.1116) radius 3.47
  circle A241 centre (9.8481, -1.7365) radius 3.47
  circle A242 centre (19.6962, -3.473) radius 3.47
  circle A243 centre (21.4326, 6.3751) radius 3.47
  circle A244 centre (23.1691, 16.2232) radius 3.47
  circle A245 centre (24.9056, 26.0713) radius 3.47
  circle A246 centre (34.7537, 24.3348) radius 3.47
  circle A247 centre (33.0172, 14.4867) radius 3.47
  circle A248 centre (31.2807, 4.6386) radius 3.47
  circle A249 centre (29.5442, -5.2094) radius 3.47
  circle A250 centre (39.3923, -6.9459) radius 3.47
  circle A251 centre (41.1288, 2.9022) radius 3.47
  circle A252 centre (42.8653, 12.7502) radius 3.47
  circle A253 centre (44.6018, 22.5983) radius 3.47
  circle A254 centre (60.1288, 22.5983) radius 3.47
  circle A255 centre (61.8653, 12.7502) radius 3.47
  circle A256 centre (63.6018, 2.9022) radius 3.47
  circle A257 centre (65.3382, -6.9459) radius 3.47
  circle A258 centre (75.1863, -5.2094) radius 3.47
  circle A259 centre (73.4498, 4.6386) radius 3.47
  circle A260 centre (71.7134, 14.4867) radius 3.47
  circle A261 centre (69.9769, 24.3348) radius 3.47
  circle A262 centre (79.8249, 26.0713) radius 3.47
  circle A263 centre (81.5614, 16.2232) radius 3.47
  circle A264 centre (83.2979, 6.3751) radius 3.47
  circle A265 centre (85.0344, -3.473) radius 3.47
  circle A266 centre (94.8825, -1.7365) radius 3.47
  circle A267 centre (93.146, 8.1116) radius 3.47
  circle A268 centre (91.4095, 17.9597) radius 3.47
  circle A269 centre (89.673, 27.8078) radius 3.47
  circle A270 centre (99.5211, 29.5442) radius 3.47
  circle A271 centre (101.2576, 19.6962) radius 3.47
  circle A272 centre (102.9941, 9.8481) radius 3.47
  circle A273 centre (104.7305, 0) radius 3.47
  constraint coincident L21.end A234
  constraint coincident L27.end A235
  constraint coincident L31.start A236
  constraint concentric A181 A237
  constraint coincident L37.start A237
  constraint concentric A185 A238
  constraint coincident L61.start A238
  constraint coincident L55.start A239
  constraint coincident L49.start A240
  constraint coincident L43.start A241
  constraint concentric A186 A242
  constraint coincident L67.start A242
  constraint coincident L73.start A243
  constraint coincident L79.start A244
  constraint concentric A189 A245
  constraint coincident L85.start A245
  constraint coincident L109.start A246
  constraint coincident L103.start A247
  constraint coincident L97.start A248
  constraint coincident L91.start A249
  constraint coincident L115.start A250
  constraint concentric A195 A251
  constraint coincident L121.start A251
  constraint coincident L127.start A252
  constraint coincident L133.start A253
  constraint coincident L253.start A254
  constraint coincident L247.start A255
  constraint coincident L241.start A256
  constraint concentric A214 A257
  constraint coincident L235.start A257
  constraint coincident L211.start A258
  constraint concentric A211 A259
  constraint coincident L217.start A259
  constraint coincident L223.start A260
  constraint concentric A213 A261
  constraint coincident L229.start A261
  constraint coincident L205.start A262
  constraint coincident L199.start A263
  constraint coincident L193.start A264
  constraint coincident L187.start A265
  constraint coincident L163.start A266
  constraint coincident L169.start A267
  constraint coincident L175.start A268
  constraint coincident L181.start A269
  constraint coincident L157.start A270
  constraint coincident L151.start A271
  constraint coincident L145.start A272
  constraint concentric A198 A273
  constraint coincident L139.start A273